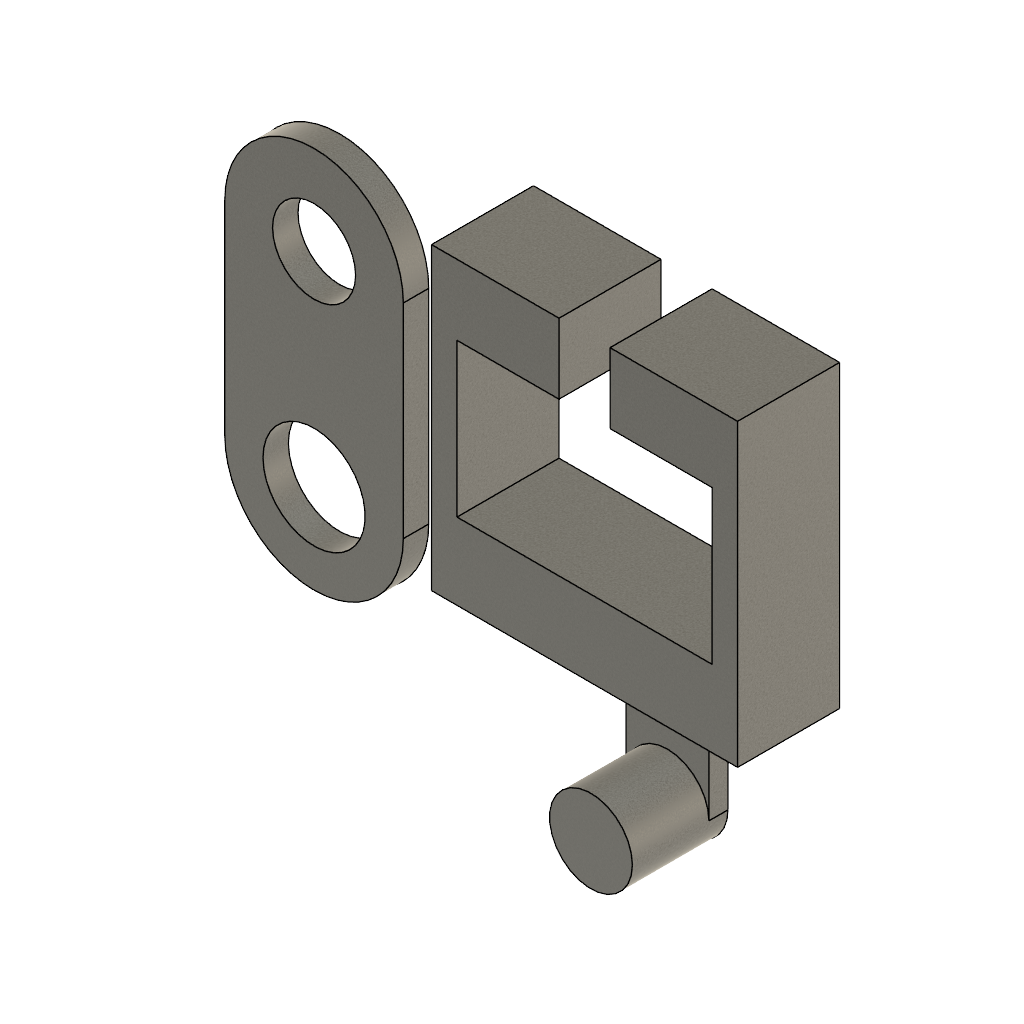
A6 (Autodesk Fusion 360 design; units mm, degrees)
part number: 2026-09-28-14-34-42-395
part number: 2026-09-28-15-31-45-336
Autodesk Fusion 360 part; units mm, degrees
sketch "Sketch1" plane through (0, 0, 0) normal (0, 1, 0) x (1, 0, 0)
  line L0 (0, 0) -> (76.2, 0)
  line L1 (76.2, 0) -> (76.2, -74.6125)
  line L2 (0, 0) -> (0, -74.6125)
  line L3 (0, -74.6125) -> (76.2, -74.6125)
  dimension "d17" = 76.2
  dimension "d18" = 74.6125
  dimension "d19" = 74.6125
  dimension "d20" = 76.2
  constraint coincident L0.start L2.start
  constraint horizontal L0
  constraint perpendicular L0 L1
  constraint perpendicular L0 L2
  constraint perpendicular L2 L3
  measures "d17" distance of L0.start L0.end
  measures "d18" distance of L0.end L1.end
  measures "d19" distance of L0.start L2.end
  measures "d20" distance of L2.end L1.end
extrude "Extrude1" add sketch "Sketch1" along normal blind 25.4 makes body 1
sketch "Sketch2" plane through (0, 0, 0) normal (0, -1, 0) x (1, 0, 0)
  line L0 (0, 74.6125) -> (0, 0)
  line L1 (0, 0) -> (76.2, 0)
  line L2 (76.2, 0) -> (76.2, 74.6125)
  line L3 (76.2, 74.6125) -> (0, 74.6125)
  line L4 (6.35, 57.15) -> (69.85, 57.15)
  line L5 (69.85, 57.15) -> (69.85, 19.05)
  line L6 (69.85, 19.05) -> (6.35, 19.05)
  line L7 (6.35, 19.05) -> (6.35, 57.15)
  dimension "d23" = 19.05
  dimension "d24" = 63.5
  dimension "d25" = 6.35
  dimension "d26" = 38.1
  constraint horizontal L4
  constraint vertical L5
  constraint horizontal L6
  constraint vertical L7
  measures "d23" distance of L1 L6
  measures "d24" distance of L5.end L6.end
  measures "d25" distance of L2 L5
  measures "d26" distance of L4.end L5.end
extrude "Extrude2" cut sketch "Sketch2" against normal through all contours L4 L5 L6 L7 bodies 1
sketch "Sketch3" plane through (0, 0, 0) normal (0, -1, 0) x (1, 0, 0)
  line L0 (6.35, 19.05) -> (6.35, 57.15)
  line L1 (6.35, 57.15) -> (69.85, 57.15)
  line L2 (69.85, 57.15) -> (69.85, 19.05)
  line L3 (69.85, 19.05) -> (6.35, 19.05)
  line L4 (0, 74.6125) -> (0, 0)
  line L5 (0, 0) -> (76.2, 0)
  line L6 (76.2, 0) -> (76.2, 74.6125)
  line L7 (76.2, 74.6125) -> (0, 74.6125)
  line L8 (31.75, 74.6125) -> (44.45, 74.6125)
  line L9 (44.45, 74.6125) -> (44.45, 57.15)
  line L10 (44.45, 57.15) -> (31.75, 57.15)
  line L11 (31.75, 57.15) -> (31.75, 74.6125)
  dimension "d28" = 12.7
  dimension "d29" = 31.75
  constraint horizontal L8
  constraint vertical L9
  constraint horizontal L10
  constraint vertical L11
  constraint coincident L1 L9.end
  constraint coincident L7 L8.start
  measures "d28" distance of L8.start L8.end
  measures "d29" distance of L4 L11
extrude "Extrude3" cut sketch "Sketch3" against normal through all contours L1 L7 L8 L9 L10 L11 bodies 1
sketch "Sketch4" plane through (0, 25.4, 0) normal (0, 1, 0) x (-1, 0, 0)
  line L0 (-31.75, 74.6125) -> (-31.75, 57.15)
  line L1 (-31.75, 57.15) -> (-6.35, 57.15)
  line L2 (-6.35, 57.15) -> (-6.35, 19.05)
  line L3 (-6.35, 19.05) -> (-69.85, 19.05)
  line L4 (-69.85, 19.05) -> (-69.85, 57.15)
  line L5 (-69.85, 57.15) -> (-44.45, 57.15)
  line L6 (-44.45, 57.15) -> (-44.45, 74.6125)
  line L7 (-44.45, 74.6125) -> (-76.2, 74.6125)
  line L8 (-76.2, 74.6125) -> (-76.2, 0)
  line L9 (-76.2, 0) -> (0, 0)
  line L10 (0, 0) -> (0, 74.6125)
  line L11 (0, 74.6125) -> (-31.75, 74.6125)
  line L12 (-48.4188, 0) -> (-27.7812, 0)
  line L13 (-27.7812, 0) -> (-27.7812, -35.7188)
  line L14 (-27.7812, -35.7188) -> (-48.4188, -35.7188)
  line L15 (-48.4188, -35.7188) -> (-48.4188, 0)
  dimension "d36" = 20.6375
  dimension "d37" = 27.7812
  dimension "d40" = 35.7188
  constraint horizontal L12
  constraint vertical L13
  constraint horizontal L14
  constraint vertical L15
  constraint coincident L9 L12.start
  measures "d36" distance of L13 L15
  measures "d37" distance of L8.end L15
  measures "d40" distance of L12.end L13.end
extrude "Extrude4" add sketch "Sketch4" against normal blind 4.7625 contours L9 L12 L13 L14 L15 bodies 1
sketch "Sketch5" plane through (0, 25.4, 0) normal (0, 1, 0) x (-1, 0, 0)
  line L0 (-31.75, 74.6125) -> (-31.75, 57.15)
  line L1 (-31.75, 57.15) -> (-6.35, 57.15)
  line L2 (-6.35, 57.15) -> (-6.35, 19.05)
  line L3 (-6.35, 19.05) -> (-69.85, 19.05)
  line L4 (-69.85, 19.05) -> (-69.85, 57.15)
  line L5 (-69.85, 57.15) -> (-44.45, 57.15)
  line L6 (-44.45, 57.15) -> (-44.45, 74.6125)
  line L7 (-44.45, 74.6125) -> (-76.2, 74.6125)
  line L8 (-76.2, 74.6125) -> (-76.2, 0)
  line L9 (-76.2, 0) -> (-48.4187, 0)
  line L10 (-48.4188, 0) -> (-48.4188, -35.7188)
  line L11 (-48.4188, -35.7188) -> (-27.7812, -35.7188)
  line L12 (-27.7812, -35.7188) -> (-27.7812, 0)
  line L13 (-27.7812, 0) -> (0, 0)
  line L14 (0, 0) -> (0, 74.6125)
  line L15 (0, 74.6125) -> (-31.75, 74.6125)
  line L16 (-27.7812, -35.7188) -> (-48.4188, -35.7188)
  circle A0 centre (-38.1, -35.7188) radius 10.3188
  dimension "d43" = 20.6375
  constraint midpoint L11 A0.centre
  measures "d43" diameter of A0
extrude "Extrude5" add sketch "Sketch5" against normal blind 23.8125 contours L11 L16 A0 | L11 L16 A0 bodies 1
sketch "Sketch1 (2)" plane through (0, 0, 0) normal (0, 1, 0) x (1, 0, 0) in component "Link"
  line L0 (-22.225, 0) -> (-22.225, -50.8)
  arc A0 (-22.225, -50.8) -> (22.225, -50.8) centre (0, -50.8) ccw
  line L1 (22.225, -50.8) -> (22.225, 0)
  arc A1 (22.225, 0) -> (-22.225, 0) centre (0, 0) ccw
  line L2 (0, 0) -> (0, -50.8) construction
  dimension "d54" = 50.8
  dimension "d55" = 44.45
  constraint tangent L0 A0
  constraint tangent A0 L1
  constraint parallel L0 L1
  constraint tangent L1 A1
  constraint tangent L0 A1
  constraint vertical L2
  constraint coincident A1.centre L2.start
  measures "d54" distance of A1.centre A0.centre
  measures "d55" distance of L0 L1
extrude "Extrude1'" add sketch "Sketch1 (2)" along normal blind 6.35 separate body makes body 2 in component "Link"
sketch "Sketch2 (2)" plane through (0, 0, 0) normal (0, -1, 0) x (1, 0, 0) in component "Link"
  arc A0 (-22.225, 0) -> (22.225, 0) centre (0, 0) ccw
  line L0 (22.225, 0) -> (22.225, 50.8)
  arc A1 (22.225, 50.8) -> (-22.225, 50.8) centre (0, 50.8) ccw
  line L1 (-22.225, 50.8) -> (-22.225, 0)
  circle A2 centre (0, 50.8) radius 10.3187
  circle A3 centre (0, 0) radius 12.7
  dimension "d58" = 20.6375
  dimension "d59" = 25.4
  constraint concentric A1 A2
  constraint coincident A0.centre A3.centre
  measures "d58" diameter of A2
  measures "d59" diameter of A3
extrude "Extrude2'" cut sketch "Sketch2 (2)" against normal blind 6.35 contours A2 | A3 bodies 2 in component "Link"
component "Link" placed x (1, 0, 0) y (0, 1, 0) z (0, 0, 1) at (-39.2785, 10.0438, -2.3292)
equation "slot_width = 0.500 in"
equation "side_recess = 1.000 in"
equation "slot_height = 1.500 in"
equation "wall_thickness = 0.250 in"
equation "bottom_thickness = ceil(c_min_thickness / size_increment) * size_increment"
equation "lip_thickness = 0.6875 in"
equation "bracket_depth = 1.000 in"
equation "opening_width = slot_width + 2 * side_recess"
equation "bracket_width = opening_width + 2 * wall_thickness"
equation "bracket_height = bottom_thickness + slot_height + lip_thickness"
equation "load_lbf = 1200"
equation "safety_factor = 4"
equation "yield_psi = 36000"
equation "c_span = opening_width + wall_thickness"
equation "size_increment = 0.0625 in"
equation "c_min_thickness = ( sqrt(( 3 * load_lbf * ( c_span / bracket_depth ) * safety_factor ) / ( 2 * yield_psi )) * 1 ) * 1 in"
equation "d17 = bracket_width"
equation "d18 = bracket_height"
equation "d19 = bracket_height"
equation "d20 = bracket_width"
equation "d21 = bracket_depth"
equation "d23 = bottom_thickness"
equation "d24 = opening_width"
equation "d25 = wall_thickness"
equation "d26 = slot_height"
equation "d28 = slot_width"
equation "d29 = ( bracket_width - slot_width ) / 2"
equation "a_diameter = 0.8125 in"
equation "b_width = 0.8125 in"
equation "b_thickness = 0.1875 in"
equation "b_clear_length = 1.000 in"
equation "b_total_length = b_clear_length + a_diameter / 2"
equation "d36 = b_width"
equation "d37 = ( bracket_width - b_width ) / 2"
equation "d38 = -b_thickness"
equation "d40 = b_total_length"
equation "a_exposed_length = 0.750 in"
equation "a_total_length = a_exposed_length + b_thickness"
equation "d43 = a_diameter"
equation "d44 = -a_total_length"
equation "link_width = 1.750 in"
equation "link_thickness = 0.250 in"
equation "link_spacing = 2.000 in"
equation "link_end_radius = link_width / 2"
equation "link_length = link_spacing + 2 * link_end_radius"
equation "link_a_hole = a_diameter"
equation "shaft_basic_diameter = 1.000 in"
equation "link_shaft_hole = shaft_basic_diameter"
equation "d54 = link_spacing"
equation "d55 = link_width"
equation "d56 = link_thickness"
equation "d58 = link_a_hole"
equation "d59 = link_shaft_hole"
equation "d60 = -link_thickness"
